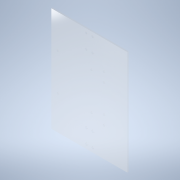
# Autodesk Inventor part: Base Plate
Saved by Autodesk Inventor 2020 (Build 240168000, 168)
## iProperties
Created: 2020-03-28
Part Number: Base Plate
Material: Polycarbonate, Clear
Document SubType Name: Modeling
Designer: Ishaan
Density: 1.2 g/cm^3
Appearance: Polycarbonate - Clear
Author: Ishaan
Autodesk Inventor part; units mm, degrees
ref_plane "YZ Plane" through (0, 0, 0) normal (1, 0, 0) x (0, 1, 0)
ref_plane "XZ Plane" through (0, 0, 0) normal (0, 1, 0) x (-1, 0, 0)
ref_plane "XY Plane" through (0, 0, 0) normal (0, 0, 1) x (1, 0, 0)
sketch "Sketch1" plane through (0, 0, 0) normal (0, 0, 1) x (1, 0, 0)
  line L0 (152.4, -209.55) -> (-152.4, -209.55)
  line L1 (-152.4, -209.55) -> (-152.4, 209.55)
  line L2 (-152.4, 209.55) -> (152.4, 209.55)
  line L3 (152.4, 209.55) -> (152.4, -209.55)
  line L4 (152.4, -209.55) -> (-152.4, 209.55) construction
  line L5 (-152.4, -209.55) -> (152.4, 209.55) construction
  line L6 (57.6, 93.25) -> (57.6, -93.25) construction
  point P0 (0, 0)
  point P1 (57.6, 55.75)
  point P2 (57.6, -55.75)
  point P3 (57.6, 0)
  point P4 (152.4, 0)
  dimension "d0" = 304.8
  dimension "d1" = 419.1
  dimension "d2" = 111.5
  dimension "d3" = 37.5
  dimension "d4" = 37.5
  dimension "d25" = 210
  constraints: 14 end point, 4 midpoint, 2 coincident, 2 parallel, 2 point on line, 1 horizontal, 1 horizontal alignment, 1 perpendicular, 1 vertical
  measures "d0" distance of L1.end L2.end
  measures "d1" distance of L0.end L1.end
  measures "d2" distance of point (57.6, -55.75) point (57.6, 55.75)
  measures "d3" distance of point (57.6, 55.75) point (57.6, 93.25)
  measures "d4" distance of point (57.6, -93.25) point (57.6, -55.75)
  measures "d25" distance between parallel lines of L6 L1
extrude "Extrusion1" add sketch "Sketch1" against normal blind 5.588
hole "Hole1" at (57.6, 55.75, 0) at (57.6, -55.75, 0) at (57.6, -93.25, 0) at (57.6, 93.25, 0) direction (0, 0, -1) diameter 7.1437 end through all
sketch "Sketch2" plane through (0, 0, 0) normal (0, 0, 1) x (1, 0, 0)
  line L0 (-127.4, 74.5) -> (7.6, 74.5) construction
  line L1 (-127.4, -74.5) -> (7.6, -74.5) construction
  circle A0 centre (57.6, 55.75) radius 3.5719 construction
  circle A1 centre (57.6, -55.75) radius 3.5719 projected
  circle A2 centre (57.6, 93.25) radius 3.5719 construction
  line L2 (57.6, 93.25) -> (57.6, 55.75) construction
  circle A3 centre (57.6, -93.25) radius 3.5719 construction
  line L3 (57.6, -93.25) -> (57.6, -55.75) construction
  point P0 (0, 0)
  point P1 (57.6, -74.5)
  point P2 (57.6, 74.5)
  dimension "d15" = 50
  dimension "d16" = 50
  dimension "d17" = 135
  constraints: 8 end point, 4 coincident, 2 horizontal, 2 midpoint, 2 point on line, 2 vertical, 1 parallel
  measures "d15" horizontal distance of L2.end point (7.6, 74.5)
  measures "d16" horizontal distance of L3.end point (7.6, -74.5)
  measures "d17" distance of L0.start L0.end
hole "Hole2" at (-127.4, 74.5, 0) at (7.6, 74.5, 0) at (7.6, -74.5, 0) at (-127.4, -74.5, 0) direction (0, 0, -1) diameter 7.1437 end through all
sketch "Sketch3" plane through (0, 0, 0) normal (0, 0, 1) x (1, 0, 0)
  line L0 (12.7, -193.675) -> (-12.7, -193.675) construction
  line L1 (-12.7, -193.675) -> (-12.7, -136.525) construction
  line L2 (-12.7, -136.525) -> (12.7, -136.525) construction
  line L3 (12.7, -136.525) -> (12.7, -193.675) construction
  line L4 (12.7, -193.675) -> (-12.7, -136.525) construction
  line L5 (-12.7, -193.675) -> (12.7, -136.525) construction
  line L6 (-12.7, 136.525) -> (12.7, 136.525) construction
  line L7 (12.7, 136.525) -> (12.7, 193.675) construction
  line L8 (12.7, 193.675) -> (-12.7, 193.675) construction
  line L9 (-12.7, 193.675) -> (-12.7, 136.525) construction
  line L10 (-12.7, 136.525) -> (12.7, 193.675) construction
  line L11 (12.7, 136.525) -> (-12.7, 193.675) construction
  line L12 (-23.8125, -202.4062) -> (23.8125, -202.4062) construction
  line L13 (23.8125, -202.4062) -> (23.8125, -127.7938) construction
  line L14 (23.8125, -127.7938) -> (-23.8125, -127.7938) construction
  line L15 (-23.8125, -127.7938) -> (-23.8125, -202.4062) construction
  line L16 (-23.8125, -202.4062) -> (23.8125, -127.7938) construction
  line L17 (23.8125, -202.4062) -> (-23.8125, -127.7938) construction
  line L18 (-23.8125, 127.7938) -> (23.8125, 127.7938) construction
  line L19 (23.8125, 127.7938) -> (23.8125, 202.4062) construction
  line L20 (23.8125, 202.4062) -> (-23.8125, 202.4062) construction
  line L21 (-23.8125, 202.4062) -> (-23.8125, 127.7938) construction
  line L22 (-23.8125, 127.7938) -> (23.8125, 202.4062) construction
  line L23 (23.8125, 127.7938) -> (-23.8125, 202.4062) construction
  line L24 (0, -165.1) -> (0, 165.1) construction
  line L25 (-152.4, -209.55) -> (152.4, -209.55) construction
  point P0 (0, 0)
  point P1 (0, 0)
  dimension "d26" = 25.4
  dimension "d27" = 57.15
  dimension "d28" = 25.4
  dimension "d29" = 57.15
  dimension "d30" = 47.625
  dimension "d31" = 74.6125
  dimension "d33" = 330.2
  constraints: 50 end point, 9 coincident, 9 midpoint, 9 parallel, 4 horizontal, 4 perpendicular, 2 equal length
  measures "d26" distance of L1.end L2.end
  measures "d27" distance of L0.end L1.end
  measures "d28" distance of L8.end L7.end
  measures "d29" distance of L7.end L6.end
  measures "d30" distance of L14.end L13.end
  measures "d31" distance of L12.end L13.end
  measures "d33" distance of L24.start L24.end
hole "Hole3" at (12.7, 193.675, 0) at (12.7, 136.525, 0) at (-12.7, 136.525, 0) at (-12.7, 193.675, 0) at (12.7, -136.525, 0) at (12.7, -193.675, 0) at (-12.7, -193.675, 0) at (-12.7, -136.525, 0) direction (0, 0, -1) diameter 8.7313 end through all
equation "\"d16\" = d15"
body "Solid1"
